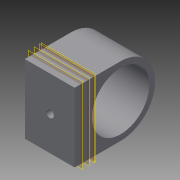
# Autodesk Inventor part: Bauteil1
Saved by Autodesk Inventor 2014 (Build 180170000, 170)
## iProperties
Created: 2014-06-16
Part Number: Bauteil1
Material: Generisch
Document SubType Name: Modeling
Designer: mdick
Density: 1 g/cm^3
Appearance: Vorgabe
Author: mdick
Autodesk Inventor part; units mm, degrees
ref_plane "YZ Plane" through (0, 0, 0) normal (1, 0, 0) x (0, 1, 0)
ref_plane "XZ Plane" through (0, 0, 0) normal (0, 1, 0) x (-1, 0, 0)
ref_plane "XY Plane" through (0, 0, 0) normal (0, 0, 1) x (1, 0, 0)
sketch "Skizze1" plane through (0, 0, 0) normal (1, 0, 0) x (0, 1, 0)
  line L0 (-21, -18) -> (21, -18)
  line L1 (21, -18) -> (21, 18)
  line L2 (21, 18) -> (-21, 18)
  line L3 (-21, 18) -> (-21, -18)
  line L4 (-21, -18) -> (21, 18) construction
  line L5 (21, -18) -> (-21, 18) construction
  point P0 (0, 0)
  dimension "d0" = 42
  dimension "d1" = 36
  constraints: 12 end point, 2 midpoint, 2 parallel, 1 horizontal, 1 perpendicular
  measures "d0" distance of L2.end L1.end
  measures "d1" distance of L1.end L0.end
extrude "Extrusion1" add sketch "Skizze1" along normal blind 26
fillet "Rundung1" radius 18 2 edges at (13, 21, 18) (13, 21, -18)
sketch "Skizze2" plane through (26, 0, 0) normal (1, 0, 0) x (0, 0, -1)
  arc A0 (18, 3) -> (-18, 3) centre (0, 3) ccw projected
  circle A1 centre (0, 3) radius 15
  point P0 (0, 0)
  dimension "d5" = 30
  constraints: 1 centre point, 1 coincident
  measures "d5" diameter of A1
hole "Bohrung1" at (26, 3, 0) direction (-1, 0, 0) diameter 30 end through all
ref_plane "Arbeitsebene2" through (0, -18, -18) normal (0, -1, 0) x (1, 0, 0)
ref_plane "Arbeitsebene3" through (0, -14.8, -18) normal (0, -1, 0) x (1, 0, 0)
sketch "Skizze3" plane through (0, -21, -18) normal (0, -1, 0) x (1, 0, 0)
  line L0 (0, 0) -> (26, 0) projected
  line L1 (3, 0) -> (23, 0)
  line L2 (23, 0) -> (23, 25)
  line L3 (23, 25) -> (3, 25)
  line L4 (3, 25) -> (3, 0)
  point P0 (0, 18)
  point P1 (13, 0)
  dimension "d15" = 20
  dimension "d16" = 25
  constraints: 8 end point, 2 midpoint, 2 parallel, 1 horizontal, 1 perpendicular
  measures "d15" distance of L3.end L2.end
  measures "d16" distance of L2.end L1.end
extrude "Extrusion2" cut sketch "Skizze3" against normal up to surface (3.2 mm away) from surface at -3
fillet "Rundung2" radius 9 2 edges at (23, -16.4, 7) (3, -16.4, 7)
ref_plane "Arbeitsebene7" through (-35.1228, -11.2, 0) normal (0, -1, 0) x (1, 0, 0)
ref_plane "Arbeitsebene6" through (-35.1228, -12, 0) normal (0, -1, 0) x (1, 0, 0)
sketch "Skizze9" plane through (-35.1228, -11.2, 0) normal (0, -1, 0) x (1, 0, 0)
  line L0 (61.1228, 15) -> (61.1228, -15) projected
  line L1 (61.1228, -18) -> (35.1228, -18) projected
  point P0 (35.1228, 0)
  point P1 (48.1228, 0)
  dimension "d49" = 13
  dimension "d50" = 18
  measures "d49" distance from line of L0 point (48.123, 0)
  measures "d50" distance from line of L1 point (48.123, 0)
hole "Bohrung5" at (13, -11.2, 0) direction (0, -1, 0) diameter 4.2 depth 15 countersink diameter 10 countersink angle 90
